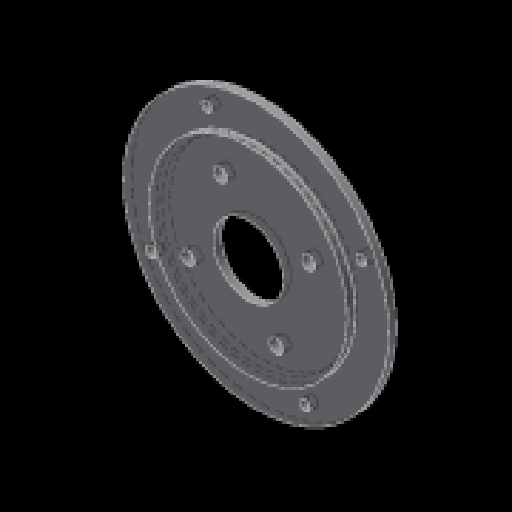
# Autodesk Inventor part: CimCoderMount
Saved by Autodesk Inventor 2025.2 (Build 292293000, 293)
## iProperties
Created: 2026-01-26
Part Number: CimCoderMount
Material: Generic
Document SubType Name: Modeling
Designer: valer
Density: 1 g/cm^3
Appearance: Default
Author: valer
Autodesk Inventor part; units mm, degrees
ref_plane "YZ Plane" through (0, 0, 0) normal (1, 0, 0) x (0, 1, 0)
ref_plane "XZ Plane" through (0, 0, 0) normal (0, 1, 0) x (-1, 0, 0)
ref_plane "XY Plane" through (0, 0, 0) normal (0, 0, 1) x (1, 0, 0)
sketch "Base" plane through (0, 0, 0) normal (0, 0, 1) x (1, 0, 0)
  circle A0 centre (0, 0) radius 50.8
  circle A1 centre (0, 0) radius 35.9875
  dimension "d0" = 101.6
  dimension "d1" = 71.975
  constraints: 2 centre point, 2 coincident
  measures "d0" diameter of A0
  measures "d1" diameter of A1
extrude "BaseFeature" add sketch "Base" along normal blind 3
ref_plane "BasePlane" through (0, 0, 0) normal (0, 0, 1) x (1, 0, 0)
sketch "EncoderMount" plane through (0, 0, 3) normal (0, 0, 1) x (1, 0, 0)
  circle A0 centre (23.0134, 10.7491) radius 2.5527 projected
  circle A1 centre (10.7491, -23.0134) radius 2.5527 projected
  circle A2 centre (-10.7491, 23.0134) radius 2.5527 projected
  line L0 (-12.5052, -15.4551) -> (-0.3296, -19.8779) projected
  line L1 (-3.9036, -29.7167) -> (-0.3296, -19.8779) projected
  arc A3 (-3.9036, -29.7167) -> (-16.0792, -25.2939) centre (0, 0) ccw construction
  line L2 (-12.5052, -15.4551) -> (-16.0792, -25.2939) projected
  circle A4 centre (-23.0134, -10.7491) radius 2.5527 projected
  circle A5 centre (-10.7491, 23.0134) radius 2.5527 projected
  circle A6 centre (23.0134, 10.7491) radius 2.5527 projected
  circle A7 centre (10.7491, -23.0134) radius 2.5527 projected
  circle A8 centre (0, 0) radius 13.335 projected
  line L3 (-1.7307, 19.0205) -> (13.5349, 13.4752) projected
  arc A9 (-2.4908, 20.6478) -> (-1.7307, 19.0205) centre (-1.2971, 20.2142) ccw projected
  line L4 (-1.19, 24.2289) -> (-2.4908, 20.6478) projected
  arc A10 (0.4373, 24.989) -> (-1.19, 24.2289) centre (0.0037, 23.7953) ccw projected
  line L5 (15.703, 19.4437) -> (0.4373, 24.989) projected
  arc A11 (16.4631, 17.8164) -> (15.703, 19.4437) centre (15.2694, 18.25) ccw projected
  line L6 (15.1622, 14.2353) -> (16.4631, 17.8164) projected
  arc A12 (13.5349, 13.4752) -> (15.1622, 14.2353) centre (13.9685, 14.6689) ccw projected
  circle A13 centre (0, 0) radius 30.48 projected
  circle A14 centre (0, 0) radius 37.9875
  circle A15 centre (0, 0) radius 35.9875 construction
  dimension "d8" = 2
  constraints: 1 centre point, 1 coincident
  measures "d8" radial gap between concentric circles of A15 A14
extrude "EncoderMountFEature" add sketch "EncoderMount" along normal blind 3 contours A9 L4 A10 L5 A11 L6 A12 L3 | A13 | A14
sketch "LegMount" plane through (0, 0, 3) normal (0, 0, 1) x (1, 0, 0)
  line L0 (0, 0) -> (18.7871, -40.2225) construction
  line L1 (-71.12, 0) -> (71.12, 0) construction
  circle A0 centre (10.7491, -23.0134) radius 2.5527 construction
  circle A1 centre (18.7871, -40.2225) radius 2
  circle A2 centre (0, 0) radius 50.8 projected
  circle A3 centre (0, 0) radius 37.9875 projected
  circle A4 centre (0, 0) radius 44.3937 construction
  circle A5 centre (-23.0134, -10.7491) radius 2.5527 projected
  line L2 (0, 0) -> (-40.2225, -18.7871) construction
  line L3 (0, 0) -> (40.2225, 18.7871) construction
  circle A6 centre (23.0134, 10.7491) radius 2.5527 construction
  circle A7 centre (-10.7491, 23.0134) radius 2.5527 construction
  line L4 (0, 0) -> (-18.7871, 40.2225) construction
  circle A8 centre (-40.2225, -18.7871) radius 2
  circle A9 centre (-18.7871, 40.2225) radius 2
  circle A10 centre (40.2225, 18.7871) radius 2
  dimension "d11" = 4
  dimension "d12" = 12.8125
  dimension "d13" = 6.4062
  dimension "d14" = 4
  dimension "d15" = 4
  dimension "d16" = 4
  constraints: 8 end point, 5 centre point, 5 coincident, 4 point on circle, 4 point on line
  measures "d11" diameter of A1
  measures "d12" radial gap between concentric circles of A2 A3
  measures "d13" radial gap between concentric circles of A2 A4
  measures "d14" diameter of A8
  measures "d15" diameter of A9
  measures "d16" diameter of A10
extrude "LegMountFeature" cut sketch "LegMount" against normal through all contours A1 | A8 | A9 | A10
equation "\"d13\" = 0.5 * d12"
equation "\"d14\" = d11"
equation "\"d15\" = d11"
equation "\"d16\" = d11"
body "Solid1"
